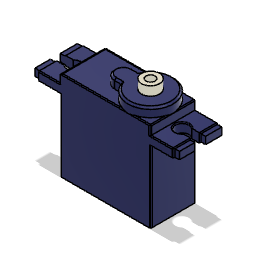
200100_Assignment_2b (Autodesk Fusion 360 design; units mm, degrees)
Autodesk Fusion 360 part; units mm, degrees
sketch "Sketch1" plane through (0, 0, 0) normal (0, 0, 1) x (1, 0, 0)
  line L0 (-50, 50) -> (50, 50)
  line L1 (50, 50) -> (50, -50)
  line L2 (50, -50) -> (-50, -50)
  line L3 (-50, -50) -> (-50, 50)
  line L4 (50, 40) -> (75, 40)
  line L5 (75, 40) -> (75, 30)
  line L6 (50, 30) -> (50, 40)
  line L7 (-50, 40) -> (-75, 40)
  line L8 (-75, 40) -> (-75, 30)
  line L9 (-75, 30) -> (-50, 30)
  line L10 (50, 30) -> (75, 30)
  dimension "d1" = 100
  dimension "d2" = 100
  dimension "d3" = 25
  dimension "d4" = 25
  dimension "d5" = 10
  dimension "d7" = 10
  constraint horizontal L0
  constraint vertical L1
  constraint horizontal L2
  constraint vertical L3
  constraint coincident L1 L4.start
  constraint perpendicular L1 L4
  constraint perpendicular L4 L5
  constraint coincident L1 L6.start
  constraint coincident L3 L7.start
  constraint perpendicular L3 L7
  constraint perpendicular L7 L8
  constraint coincident L3 L9.end
  constraint perpendicular L3 L9
  constraint perpendicular L5 L10
  measures "d1" distance of L0.start L0.end
  measures "d2" distance of L0.end L1.end
  measures "d3" distance of L7.start L7.end
  measures "d4" distance of L4.start L4.end
  measures "d5" distance of L0.start L7.start
  measures "d7" distance of L7.end L8.end
extrude "Extrude1" add sketch "Sketch1" along normal blind 25 and the other way blind 25
sketch "Sketch2" plane through (0, 0, 25) normal (0, 0, 1) x (1, 0, 0)
  line L0 (50, -50) -> (50, 30)
  line L1 (50, 30) -> (75, 30)
  line L2 (75, 30) -> (75, 40)
  line L3 (75, 40) -> (50, 40)
  line L4 (50, 40) -> (50, 50)
  line L5 (50, 50) -> (-50, 50)
  line L6 (-50, 50) -> (-50, 40)
  line L7 (-50, 40) -> (-75, 40)
  line L8 (-75, 40) -> (-75, 30)
  line L9 (-75, 30) -> (-50, 30)
  line L10 (-50, 30) -> (-50, -50)
  line L11 (-50, -50) -> (50, -50)
sketch "Sketch3" plane through (0, 50, 0) normal (0, 1, 0) x (-1, 0, 0)
  line L0 (50, -25) -> (50, 25)
  line L1 (50, 25) -> (-50, 25)
  line L2 (-50, 25) -> (-50, -25)
  line L3 (-50, -25) -> (50, -25)
  circle A0 centre (-25, 0) radius 25
  line L4 (5, -10) -> (-2.0871, -10)
  line L5 (5, 10) -> (-2.0871, 10)
  arc A1 (5, -10) -> (5, 10) centre (5, 0) ccw
  circle A2 centre (-25, 0) radius 10
  circle A3 centre (-25, 0) radius 5
  circle A4 centre (60, 0) radius 7.5
  circle A5 centre (-60, 0) radius 7.5
  line L6 (75, -5) -> (65.5902, -5)
  line L7 (75, 5) -> (65.5902, 5)
  line L8 (65.5902, 5) -> (75, 5)
  line L9 (-75, -5) -> (-65.5902, -5)
  line L10 (-75, 5) -> (-65.5902, 5)
  line L11 (75, -5) -> (75, 5)
  line L12 (-75, -5) -> (-75, 5)
  point P0 (75, 25)
  point P1 (-75, -25)
  point P2 (75, -25)
  dimension "d14" = 7.0871
  dimension "d15" = 10
  dimension "d16" = 20
  dimension "d17" = 10
  dimension "d18" = 15
  dimension "d19" = 15
  dimension "d25" = 9.4098
  dimension "d27" = 20
  dimension "d28" = 10
  dimension "d29" = 9.4098
  constraint tangent L2 A0
  constraint coincident A0 L4.end
  constraint parallel L3 L4
  constraint coincident A0 L5.end
  constraint perpendicular L0 L5
  constraint tangent L4 A1
  constraint tangent L5 A1
  constraint concentric A0 A2
  constraint concentric A0 A3
  constraint coincident A4 L6.end
  constraint horizontal L6
  constraint coincident A4 L7.end
  constraint parallel L6 L7
  constraint coincident A5 L9.end
  constraint horizontal L9
  constraint coincident A5 L10.end
  constraint parallel L9 L10
  measures "d14" distance of L4.start L4.end
  measures "d15" radius of A1
  measures "d16" diameter of A2
  measures "d17" diameter of A3
  measures "d18" diameter of A4
  measures "d19" diameter of A5
  measures "d25" distance of L9.start L9.end
  measures "d27" distance of L6.start P2
  measures "d28" distance of L6.start L7.start
  measures "d29" distance of L6.start L6.end
extrude "Extrude2" cut sketch "Sketch3" against normal blind 20 contours A4 | A4 L6 L7 L8 L11 | A5 | A5 L9 L10 L12
extrude "Extrude3" add sketch "Sketch3" along normal blind 20 contours A2
extrude "Extrude4" add sketch "Sketch3" along normal blind 10 contours A0
extrude "Extrude5" add sketch "Sketch3" along normal blind 10 contours A0 L4 L5 A1
chamfer "Chamfer1" distance 2 angle 45 4 edges at (-15, 60, 0) (-1.4564, 60, 10) (-1.4564, 60, -10) (50, 60, 0)
chamfer "Chamfer2" distance 1 angle 45 7 edges at (-50, 50, 0) (-12.5, 50, 25) (-12.5, 50, -25) (37.5, 50, -25) (50, 50, -12.5) (50, 50, 12.5) (37.5, 50, 25)
chamfer "Chamfer3" distance 1 angle 45 10 edges at (50, -10, 25) (50, 44.5, 25) (62.5, 40, 25) (75, 35, 25) (62.5, 30, 25) (0, -50, 25) (-50, -10, 25) (-62.5, 30, 25) (-62.5, 40, 25) (-75, 35, 25)
chamfer "Chamfer4" distance 1 angle 45 11 edges at (52.5, 40, 0) (75, 35, -5) (75, 40, -15) (75, 30, -15) (75, 35, 5) (75, 35, -25) (50, 44.5, -25) (49, 44, 25) (50, -10, 24) (50, -10, -25) (50, -50, -0.5) 1 faces at (75, 36.6667, 11.3333)
chamfer "Chamfer5" distance 1 angle 45 2 edges at (-49, 50, 0) (-15.5, 50, -24)
chamfer "Chamfer6" distance 1 angle 45 4 edges at (61.5, 40, -25) (61.5, 30, -25) (-62.5, 40, -25) (-62.5, 30, -25)
chamfer "Chamfer7" distance 1 angle 45 2 edges at (-50, -9.5, -25) (-0.5, -50, -25)
chamfer "Chamfer8" distance 1 angle 45 3 edges at (-75, 35, -25) (-75, 30, -14.5) (-75, 40, -14.5)
chamfer "Chamfer9" distance 1 angle 45 4 edges at (-75, 35, 5) (-75, 30, 14.5) (-75, 35, 24) (-75, 40, 14.5)
chamfer "Chamfer10" distance 1 angle 45 1 edges at (-50, -50, 0)
extrude "Extrude6" add 2 faces at (75, 36.3333, 11.6667) (75, 36.3333, -18) along direction (1, 0, 0) blind 5
extrude "Extrude7" add 2 faces at (-75, 36.3333, 11.6667) (-75, 36.3333, -17.6667) along direction (-1, 0, 0) blind 5
named bodies: "200100_Body"
